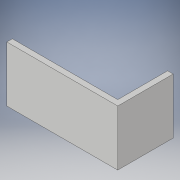
# Autodesk Inventor part: lift box
Saved by Autodesk Inventor 2019 (Build 230136000, 136)
## iProperties
Created: 2018-10-02
Part Number: lift box
Material: Generic
Document SubType Name: Modeling
Designer: User
Density: 1 g/cm^3
Appearance: Default
Author: User
Autodesk Inventor part; units mm, degrees
ref_plane "YZ Plane" through (0, 0, 0) normal (1, 0, 0) x (0, 1, 0)
ref_plane "XZ Plane" through (0, 0, 0) normal (0, 1, 0) x (-1, 0, 0)
ref_plane "XY Plane" through (0, 0, 0) normal (0, 0, 1) x (1, 0, 0)
sketch "Sketch1" plane through (0, 0, 0) normal (0, 1, 0) x (-1, 0, 0)
  line L0 (0, 0) -> (-152.4, 0)
  line L1 (-152.4, 0) -> (-152.4, -76.2)
  line L2 (-152.4, -76.2) -> (0, -76.2)
  line L3 (0, -76.2) -> (0, 0)
  dimension "d0" = 152.4
  dimension "d1" = 76.2
  constraints: 8 end point, 2 parallel, 1 horizontal, 1 perpendicular
  measures "d0" distance of L2.end L1.end
  measures "d1" distance of L1.end L0.end
extrude "Extrusion1" add sketch "Sketch1" along normal blind 76.2
shell "Shell1" thickness 7.62 removed faces 1 at (101.6, 76.2, -25.4)
sketch "Sketch2" plane through (0, 0, -76.2) normal (-1, 0, 0) x (0, 0, 1)
  line L0 (0, 0) -> (0, 76.2) projected
  line L1 (0, 76.2) -> (68.58, 76.2)
  line L2 (68.58, 76.2) -> (68.58, 7.62)
  line L3 (68.58, 7.62) -> (0, 7.62)
  line L4 (0, 7.62) -> (0, 76.2)
  line L5 (0, 0) -> (76.2, 0) projected
  line L6 (76.2, 0) -> (76.2, 76.2) projected
  point P0 (7.62, 76.2)
  dimension "d5" = 7.62
  dimension "d6" = 7.62
  dimension "d7" = 7.62
  constraints: 8 end point, 2 parallel, 1 horizontal, 1 perpendicular
  measures "d5" distance of L0.end point (7.62, 76.2)
  measures "d6" distance between parallel lines of L5 L3
  measures "d7" distance between parallel lines of L6 L2
extrude "Extrusion2" cut sketch "Sketch2" against normal up to surface (144.78 mm away)
sketch "Sketch3" plane through (0, 7.62, -7.62) normal (0, 1, 0) x (1, 0, 0)
  circle A0 centre (12.7, 11.43) radius 3.175
  line L0 (0, 0) -> (0, 68.58) projected
  line L1 (0, -7.62) -> (152.4, -7.62) projected
  dimension "d10" = 6.35
  dimension "d11" = 12.7
  dimension "d12" = 19.05
  constraints: 1 centre point
  measures "d10" diameter of A0
  measures "d11" distance from line of L0 A0.centre
  measures "d12" distance from line of A0.centre L1
extrude "Extrusion3" cut sketch "Sketch3" against normal blind 25.4
body "Solid1"
